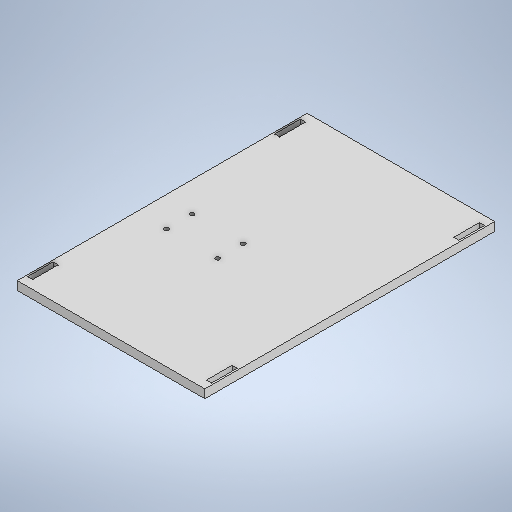
# Autodesk Inventor part: châssis haut avant
Saved by Autodesk Inventor 2026.2 (Build 302298010, 298A)
## iProperties
Created: 2026-04-15
Part Number: châssis haut avant
Material: Générique
Document SubType Name: Modeling
Designer: Genon
Density: 1 g/cm^3
Appearance: Par défaut
Author: Genon
Autodesk Inventor part; units mm, degrees
ref_plane "YZ Plane" through (0, 0, 0) normal (1, 0, 0) x (0, 1, 0)
ref_plane "XZ Plane" through (0, 0, 0) normal (0, 1, 0) x (-1, 0, 0)
ref_plane "XY Plane" through (0, 0, 0) normal (0, 0, 1) x (1, 0, 0)
sketch "Esquisse1" plane through (0, 0, 0) normal (0, 1, 0) x (-1, 0, 0)
  line L0 (0, 0) -> (110, 0)
  line L1 (110, 0) -> (110, -170)
  line L2 (110, -170) -> (0, -170)
  line L3 (0, -170) -> (0, 0)
  dimension "d0" = 110
  dimension "d1" = 170
  constraints: 8 end point, 2 parallel, 1 horizontal, 1 perpendicular
  measures "d0" distance of L1.end L2.end
  measures "d1" distance of L0.end L1.end
extrude "Extrusion1" add sketch "Esquisse1" along normal blind 5
sketch "Esquisse2" plane through (0, 5, 0) normal (0, 1, 0) x (1, 0, 0)
  line L0 (-110, 0) -> (0, 0) projected
  line L1 (-110, 0) -> (-110, 5)
  line L2 (-110, 170) -> (-110, 0) projected
  line L3 (-110, 5) -> (-105, 5)
  line L4 (-105, 5) -> (-106, 5)
  line L5 (-106, 5) -> (-106, 20)
  line L6 (-106, 20) -> (-109, 20)
  line L7 (-109, 20) -> (-109, 5)
  line L8 (-55, 0) -> (-55, 170)
  line L9 (-55, 85) -> (-68.7933, 85)
  line L10 (0, 5) -> (-5, 5)
  line L11 (-4, 5) -> (-4, 20)
  line L12 (-4, 20) -> (-1, 20)
  line L13 (-1, 20) -> (-1, 5)
  line L14 (-110, 165) -> (-105, 165)
  line L15 (-106, 165) -> (-106, 150)
  line L16 (-106, 150) -> (-109, 150)
  line L17 (-109, 150) -> (-109, 165)
  line L18 (-4, 165) -> (-4, 150)
  line L19 (-1, 150) -> (-1, 165)
  line L20 (0, 165) -> (-5, 165)
  line L21 (-4, 150) -> (-1, 150)
  dimension "d4" = 5
  dimension "d5" = 5
  dimension "d6" = 1
  dimension "d7" = 15
  dimension "d8" = 3
  dimension "d9" = 90
  dimension "d10" = 13.7933
  dimension "d11" = 85
  constraints: 40 end point, 18 symmetric about line, 9 point on line, 3 midpoint, 3 perpendicular, 2 horizontal, 1 vertical
  measures "d4" distance of L0.start L1.end
  measures "d5" distance of L1.end L3.end
  measures "d6" distance of L3.end L4.end
  measures "d7" distance of L4.end L5.end
  measures "d8" distance of L5.end L6.end
  measures "d9" angle of L8 L9
  measures "d10" distance of L9.start L9.end
  measures "d11" distance of point (-55, 0) L9.start
extrude "Extrusion2" cut sketch "Esquisse2" against normal blind 5
sketch "Esquisse3" plane through (0, 5, 0) normal (0, 1, 0) x (1, 0, 0)
  line L0 (-110, 0) -> (0, 0) projected
  line L1 (-110, 0) -> (-110, 70)
  line L2 (-110, 170) -> (-110, 0) projected
  line L3 (-110, 70) -> (-92.5, 70)
  line L4 (-92.5, 70) -> (-92.5, 85)
  line L5 (-92.5, 85) -> (-62.5, 85)
  line L6 (-62.5, 85) -> (-62.5, 70)
  dimension "d14" = 70
  dimension "d15" = 17.5
  dimension "d16" = 15
  dimension "d17" = 30
  constraints: 10 end point, 4 coincident, 2 perpendicular, 1 horizontal, 1 point on line, 1 vertical
  measures "d14" distance of L0.start L1.end
  measures "d15" distance of L1.end L3.end
  measures "d16" distance of L4.start L4.end
  measures "d17" distance of L4.end L5.end
hole "Perçage1" at (-92.5, 5, -70) at (-92.5, 5, -85) at (-62.5, 5, -85) at (-62.5, 5, -70) direction (0, -1, 0) diameter 2.459 end through all thread size "M3x0.5" class "6H" standard "ISO Metric profile"
